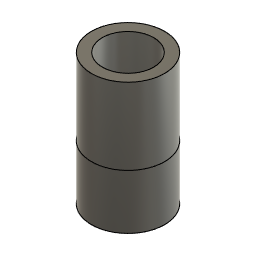
DC to Lego Coupler_ (Autodesk Fusion 360 design; units mm, degrees)
Autodesk Fusion 360 part; units mm, degrees
sketch "Sketch1" plane through (0, 0, 0) normal (0, 1, 0) x (1, 0, 0)
  circle A0 centre (0, 0) radius 1.05
  circle A1 centre (0, 0) radius 2.35
  circle A2 centre (0, 0) radius 3.35
  circle A3 centre (0, 0) radius 1.55
  dimension "d1" = 2.1
  dimension "d2" = 4.7
  dimension "d5" = 1
  dimension "d6" = 0.5
  constraint coincident A0.centre A1.centre
  measures "d1" diameter of A0
  measures "d2" diameter of A1
extrude "Extrude4" add sketch "Sketch1" along normal blind 5 contours A1 | A2 | A3 makes body 1
extrude "Extrude3" add sketch "Sketch1" along normal blind 12 separate body contours A2 makes body 2
